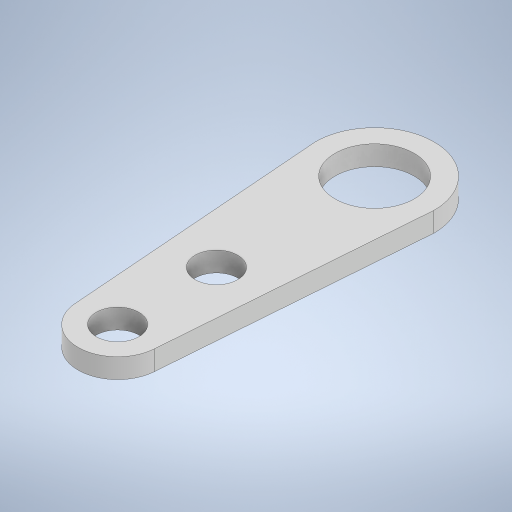
# Autodesk Inventor part: servoya giden parca
Saved by Autodesk Inventor 2023 (Build 270158000, 158)
## iProperties
Created: 2023-02-07
Part Number: servoya giden parca
Material: Generic
Document SubType Name: Modeling
Designer: omuru
Density: 1 g/cm^3
Appearance: Default
Author: omuru
Autodesk Inventor part; units mm, degrees
ref_plane "YZ Plane" through (0, 0, 0) normal (1, 0, 0) x (0, 1, 0)
ref_plane "XZ Plane" through (0, 0, 0) normal (0, 1, 0) x (-1, 0, 0)
ref_plane "XY Plane" through (0, 0, 0) normal (0, 0, 1) x (1, 0, 0)
sketch "Sketch1" plane through (0, 0, 0) normal (0, 1, 0) x (-1, 0, 0)
  arc A0 (-2.9651, 0.4562) -> (2.9651, 0.4562) centre (0, 0) ccw
  line L0 (0, 0) -> (0, 8)
  circle A1 centre (0, 8) radius 1.075
  line L1 (0, 8) -> (0, 13)
  circle A2 centre (0, 13) radius 1.075
  arc A3 (1.9942, 13.1525) -> (-1.9942, 13.1525) centre (0, 13) ccw
  line L2 (3, 0) -> (1.9942, 13.1525)
  line L3 (-3, 0) -> (-1.9942, 13.1525)
  circle A4 centre (0, 0) radius 2
  dimension "d0" = 6
  dimension "d1" = 8
  dimension "d2" = 2.15
  dimension "d3" = 5
  dimension "d4" = 2.15
  dimension "d5" = 4
  dimension "d6" = 4
  constraints: 8 end point, 6 point on circle, 5 centre point, 5 coincident, 2 point on line, 2 tangent, 2 vertical
  measures "d0" diameter of A0
  measures "d1" distance of L0.start L0.end
  measures "d2" diameter of A1
  measures "d3" distance of L1.start L1.end
  measures "d4" diameter of A2
  measures "d5" diameter of A3
  measures "d6" diameter of A4
extrude "Extrusion1" add sketch "Sketch1" against normal blind 1 contours L3 A3 L2 A0
body "Solid1"
